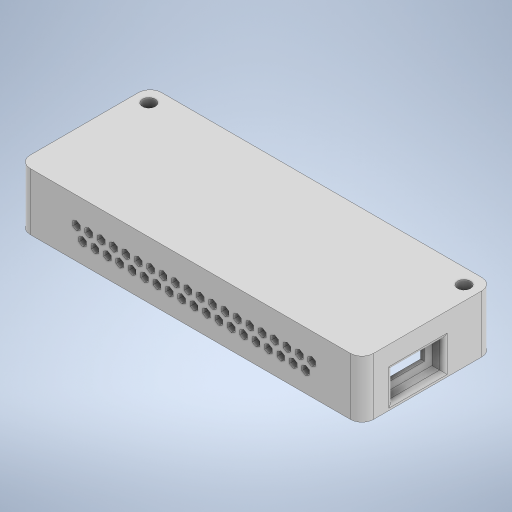
# Autodesk Inventor part: esp32_mount
Saved by Autodesk Inventor 2024 (Build 280153000, 153)
## iProperties
Created: 2024-01-28
Part Number: esp32_mount
Material: Generic
Document SubType Name: Modeling
Designer: crow
Density: 1 g/cm^3
Appearance: Default
Author: crow
## iProperties of the stored document esp32_mount_3DPrint.ipt
Created: 2024-01-28
Part Number: esp32_mount_3DPrint
Material: Generic
Document SubType Name: Modeling
Designer: crow
Density: 1 g/cm^3
Appearance: Default
Author: crow
Autodesk Inventor part; units mm, degrees
ref_plane "YZ Plane" through (0, 0, 0) normal (1, 0, 0) x (0, 1, 0)
ref_plane "XZ Plane" through (0, 0, 0) normal (0, 1, 0) x (-1, 0, 0)
ref_plane "XY Plane" through (0, 0, 0) normal (0, 0, 1) x (1, 0, 0)
sketch "Sketch1" plane through (0, 0, 0) normal (0, 1, 0) x (-1, 0, 0)
  line L0 (-0.1447, 76.4776) -> (-0.1447, -67.7737) construction
  line L1 (44.8553, -21.2084) -> (-45.1447, -21.2084)
  line L2 (-45.1447, -21.2084) -> (-45.1447, -13.2084)
  line L3 (-45.1447, -13.2084) -> (44.8553, -13.2084)
  line L4 (44.8553, -13.2084) -> (44.8553, -21.2084)
  line L5 (40.8553, 10.2416) -> (-41.1447, 10.2416)
  line L6 (-41.1447, 10.2416) -> (-41.1447, -13.2084)
  line L7 (-41.1447, -13.2084) -> (40.8553, -13.2084)
  line L8 (40.8553, -13.2084) -> (40.8553, 10.2416)
  circle A0 centre (8.6753, 7.4066) radius 1.25
  circle A1 centre (8.6753, -10.3734) radius 1.25
  circle A2 centre (-37.0447, -10.3734) radius 1.25
  line L9 (8.6753, 7.4066) -> (8.6753, -10.3734) construction
  line L10 (40.8553, -13.2084) -> (44.8553, -13.2084)
  line L11 (44.8553, -13.2084) -> (44.8553, 13.2416)
  line L12 (44.8553, 13.2416) -> (40.8553, 13.2416)
  line L13 (40.8553, 13.2416) -> (40.8553, -13.2084)
  line L14 (40.8553, 13.2416) -> (-45.1447, 13.2416)
  line L15 (-45.1447, 13.2416) -> (-45.1447, -13.2084)
  circle A3 centre (-37.0447, 7.4066) radius 1.25
  line L16 (-47.1247, -1.4834) -> (-6.1707, -1.4834) construction
  point P0 (0, 0)
  point P1 (41.1603, -17.2084)
  point P2 (-41.4497, -17.2084)
  point P3 (-0.1447, -13.2084)
  point P4 (8.6753, -1.4834)
  point P5 (40.8553, -13.2084)
  dimension "d0" = 82.61
  dimension "d1" = 41.305
  dimension "d2" = 90
  dimension "d3" = 8
  dimension "d4" = 4
  dimension "d5" = 3.695
  dimension "d6" = 82
  dimension "d7" = 23.45
  dimension "d10" = 2.5
  dimension "d11" = 17.78
  dimension "d16" = 43.22
  dimension "d17" = 4
  dimension "d18" = 3
  dimension "d19" = 4
  dimension "d82" = 2.5
  dimension "d85" = 4.1
  dimension "d86" = 45.72
  dimension "d87" = 17.78
  dimension "d91" = 11.725
  dimension "d92" = 8.89
  constraints: 34 end point, 6 parallel, 5 horizontal, 4 centre point, 4 perpendicular, 3 midpoint, 2 equal radius, 2 point on line, 2 vertical
  measures "d0" distance of point (41.16, -17.208) point (-41.45, -17.208)
  measures "d1" distance from line of L0 point (-41.45, -17.208)
  measures "d2" distance of L2.end L3.end
  measures "d3" distance of L1.end L2.end
  measures "d4" distance from line of L1 point (-41.45, -17.208)
  measures "d5" distance from line of L2 point (-41.45, -17.208)
  measures "d6" distance of L7.end L6.end
  measures "d7" distance of L6.end L5.end
  measures "d10" diameter of A0
  measures "d11" distance of L9.end L9.start
  measures "d17" distance of L12.end L11.end
  measures "d18" distance between parallel lines of L5 L12
  measures "d19" distance between parallel lines of L6 L15
  measures "d82" diameter of A3
  measures "d85" distance from line of L6 A3.centre
  measures "d86" distance of L9.start A3.centre
  measures "d87" distance of A2.centre A3.centre
  measures "d91" distance between parallel lines of L7 L16
  measures "d92" distance from line of L16 A2.centre
extrude "Extrusion1" add sketch "Sketch1" along normal blind 15 contours L1 L2 L3 L4 | L3 L8 L13 L12 L11 | L15 L14 L13 L5 L6 L3
sketch "Sketch2" plane through (0, 15, 0) normal (0, 1, 0) x (1, 0, 0)
  line L0 (-44.8553, 21.2084) -> (-44.8553, -13.2416) construction
  line L1 (45.1447, -13.2416) -> (45.1447, 21.2084) construction
  line L2 (50.5404, 17.2084) -> (-51.1103, 17.2084) construction
  point P0 (0, 0)
  point P1 (-41.1603, 17.2084)
  point P2 (41.4497, 17.2084)
  point P3 (-44.8553, 13.2084)
  point P4 (45.1447, 13.2084)
  dimension "d22" = 82.61
  dimension "d23" = 3.695
  constraints: 2 end point, 2 horizontal, 1 point on line
  measures "d22" distance of point (-41.16, 17.208) point (41.45, 17.208)
  measures "d23" distance from line of L1 point (41.45, 17.208)
hole "Hole1" at (-41.1603, 15, -17.2084) at (41.4497, 15, -17.2084) direction (0, -1, 0) diameter 3.4 depth 15 clearance for "Countersunk Flat Head Screw ISO 2009/7046" size "M3" standard "ISO"
sketch "Sketch3" plane through (0, 15, 0) normal (0, 1, 0) x (1, 0, 0)
  line L0 (45.1447, 21.2084) -> (-44.8553, 21.2084) projected
  line L1 (-40.8553, 13.2084) -> (41.1447, 13.2084) projected
  line L2 (-44.8553, 21.2084) -> (-29.4803, 21.2084)
  line L3 (-29.4803, 21.2084) -> (-29.4803, 13.2084)
  line L4 (-29.4803, 13.2084) -> (-44.8553, 13.2084)
  line L5 (-44.8553, 13.2084) -> (-44.8553, 21.2084)
  line L6 (-40.8553, 13.2084) -> (41.1447, 13.2084) projected
  line L7 (45.1447, -13.2416) -> (45.1447, 21.2084) projected
  line L8 (29.7697, 13.2084) -> (45.1447, 13.2084)
  line L9 (45.1447, 13.2084) -> (45.1447, 21.2084)
  line L10 (45.1447, 21.2084) -> (29.7697, 21.2084)
  line L11 (29.7697, 21.2084) -> (29.7697, 13.2084)
  circle A0 centre (-41.1603, 17.2084) radius 1.7 projected
  circle A1 centre (-41.1603, 17.2084) radius 3.1
  circle A2 centre (41.4497, 17.2084) radius 1.7 projected
  circle A3 centre (41.4497, 17.2084) radius 3.1
  point P0 (0, 0)
  point P1 (-44.8553, 13.2084)
  point P2 (45.1447, 13.2084)
  point P3 (-44.8553, 13.2084)
  point P4 (-40.8553, 5.069)
  point P5 (-40.8553, 2.0977)
  dimension "d72" = 1.4
  dimension "d73" = 1.4
  constraints: 16 end point, 4 parallel, 2 centre point, 2 coincident, 2 horizontal, 2 perpendicular, 1 other
  measures "d73" radial gap between concentric circles of A3 A2
extrude "Extrusion2" [suppressed]
sketch "Sketch4" plane through (0, 15, 0) normal (0, 1, 0) x (1, 0, 0)
  line L0 (41.1447, -10.2416) -> (-40.8553, -10.2416) projected
  line L1 (41.1447, 13.2084) -> (41.1447, -10.2416) projected
  line L2 (-40.8553, -10.2416) -> (41.1447, -10.2416)
  line L3 (41.1447, -10.2416) -> (41.1447, 13.2084)
  line L4 (41.1447, 13.2084) -> (-40.8553, 13.2084)
  line L5 (-40.8553, 13.2084) -> (-40.8553, -10.2416)
  point P0 (0, 0)
  constraints: 8 end point, 2 parallel, 1 horizontal, 1 perpendicular
extrude "Extrusion3" add sketch "Sketch4" against normal blind 2
sketch "Sketch5" plane through (0, 13, 0) normal (0, -1, 0) x (1, 0, 0)
  circle A0 centre (37.0447, -10.3734) radius 1.25 projected
  circle A1 centre (-8.6753, -10.3734) radius 1.25 projected
  circle A2 centre (-8.6753, 7.4066) radius 1.25 projected
  circle A3 centre (-8.6753, 7.4066) radius 2.5
  circle A4 centre (-8.6753, -10.3734) radius 2.5
  circle A5 centre (37.0447, -10.3734) radius 2.5
  circle A6 centre (37.0447, 7.4066) radius 1.25 projected
  circle A7 centre (37.0447, 7.4066) radius 2.5
  point P0 (0, 0)
  dimension "d35" = 5
  dimension "d36" = 5
  dimension "d37" = 5
  dimension "d83" = 5
  constraints: 4 centre point, 4 coincident
  measures "d35" diameter of A3
  measures "d36" diameter of A4
  measures "d37" diameter of A5
  measures "d83" diameter of A7
extrude "Extrusion4" add sketch "Sketch5" along normal blind 5 contours A0 | A1 | A2 | A3 | A4 | A5 | A6 | A7
sketch "Sketch6" plane through (37.0447, 8, -10.3734) normal (0, -1, 0) x (1, 0, 0)
  circle A0 centre (0, 0) radius 2.5 projected
  circle A1 centre (-45.72, 17.78) radius 2.5 projected
  circle A2 centre (-45.72, 0) radius 2.5 projected
  circle A3 centre (0, 17.78) radius 2.5 projected
  point P0 (-37.0447, 10.3734)
  point P1 (-45.72, 17.78)
  point P2 (-45.72, 0)
  point P3 (0, 17.78)
  constraints: 4 coincident
hole "Hole2" at (37.0447, 8, -10.3734) at (-8.6753, 8, 7.4066) at (-8.6753, 8, -10.3734) at (37.0447, 8, 7.4066) direction (0, 1, 0) diameter 2.4 depth 5
sketch "Sketch7" plane through (45.1447, 0, -14.0084) normal (-1, 0, 0) x (0, 0, 1)
  line L0 (7.885, 3.54) -> (17.225, 3.54)
  line L1 (17.225, 3.54) -> (17.225, 6.95)
  line L2 (17.225, 6.95) -> (7.885, 6.95)
  line L3 (7.885, 6.95) -> (7.885, 3.54)
  line L4 (0, 0) -> (27.25, 0) projected
  line L5 (0, 0) -> (0, 5) projected
  line L6 (27.25, 0) -> (27.25, 15) projected
  line L7 (0.8, 0) -> (0.8, 13) projected
  line L8 (27.25, 0) -> (-7.2, 0) projected
  point P0 (14.0084, 0)
  point P1 (24.25, 0)
  dimension "d53" = 6.95
  dimension "d56" = 7.025
  dimension "d88" = 7.085
  dimension "d89" = 3.54
  constraints: 8 end point, 2 parallel, 1 horizontal, 1 perpendicular, 1 other
  measures "d53" distance between parallel lines of L4 L2
  measures "d56" distance from line of point (24.25, 0) L1
  measures "d89" distance between parallel lines of L4 L0
extrude "Extrusion5" cut sketch "Sketch7" along normal blind 5
sketch "Sketch8" plane through (45.1447, 0, -14.0084) normal (-1, 0, 0) x (0, 0, 1)
  line L0 (5.885, 1.54) -> (19.225, 1.54)
  line L1 (19.225, 1.54) -> (19.225, 8.95)
  line L2 (19.225, 8.95) -> (5.885, 8.95)
  line L3 (5.885, 8.95) -> (5.885, 1.54)
  line L4 (7.885, 3.54) -> (17.225, 3.54) projected
  line L5 (7.885, 6.95) -> (7.885, 3.54) projected
  line L6 (17.225, 6.95) -> (7.885, 6.95) projected
  line L7 (17.225, 3.54) -> (17.225, 6.95) projected
  point P0 (14.0084, 0)
  dimension "d93" = 2
  dimension "d94" = 2
  dimension "d95" = 2
  dimension "d96" = 2
  constraints: 8 end point, 2 parallel, 1 horizontal, 1 perpendicular
  measures "d93" distance between parallel lines of L5 L3
  measures "d94" distance between parallel lines of L0 L4
  measures "d95" distance between parallel lines of L1 L7
  measures "d96" distance between parallel lines of L6 L2
extrude "Extrusion6" cut sketch "Sketch8" along normal blind 3 contours L3 L2 L1 L0 | L5 L6 L7 L4
fillet "Fillet2" radius 1 4 edges at (45.1447, 5.245, -8.1234) (45.1447, 1.54, -1.4534) (45.1447, 8.95, -1.4534) (45.1447, 5.245, 5.2166)
sketch "Sketch9" plane through (-44.8553, 0, 13.2416) normal (0, 0, 1) x (1, 0, 0)
  line L0 (39.5056, 7.1579) -> (41.1292, 6.2205)
  line L1 (41.1292, 6.2205) -> (41.1292, 4.3457)
  line L2 (41.1292, 4.3457) -> (39.5056, 3.4083)
  line L3 (39.5056, 3.4083) -> (37.882, 4.3457)
  line L4 (37.882, 4.3457) -> (37.882, 6.2205)
  line L5 (37.882, 6.2205) -> (39.5056, 7.1579)
  line L6 (39.5056, 7.1579) -> (39.5056, 9.0326)
  line L7 (39.5056, 9.0326) -> (37.882, 9.97)
  line L8 (37.882, 9.97) -> (36.2584, 9.0326)
  line L9 (36.2584, 9.0326) -> (36.2584, 7.1579)
  line L10 (36.2584, 7.1579) -> (37.882, 6.2205)
  line L11 (37.882, 6.2205) -> (37.882, 4.3457)
  line L12 (34.6348, 4.3457) -> (34.6348, 6.2205)
  line L13 (36.2584, 3.4083) -> (34.6348, 4.3457)
  line L14 (37.882, 4.3457) -> (36.2584, 3.4083)
  line L15 (34.6348, 6.2205) -> (36.2584, 7.1579)
  line L16 (34.6348, 9.97) -> (36.2584, 9.0326)
  line L17 (36.2584, 7.1579) -> (36.2584, 9.0326)
  line L18 (34.6348, 9.97) -> (33.0112, 9.0326)
  line L19 (33.0112, 9.0326) -> (33.0112, 7.1579)
  line L20 (33.0112, 7.1579) -> (34.6348, 6.2205)
  line L21 (33.0112, 3.4083) -> (34.6348, 4.3457)
  line L22 (34.6348, 6.2205) -> (34.6348, 4.3457)
  line L23 (31.3876, 4.3457) -> (31.3876, 6.2205)
  line L24 (31.3876, 4.3457) -> (33.0112, 3.4083)
  line L25 (31.3876, 6.2205) -> (33.0112, 7.1579)
  line L26 (31.3876, 9.97) -> (33.0112, 9.0326)
  line L27 (33.0112, 7.1579) -> (33.0112, 9.0326)
  line L28 (29.764, 7.1579) -> (29.764, 9.0326)
  line L29 (29.764, 7.1579) -> (31.3876, 6.2205)
  line L30 (29.764, 9.0326) -> (31.3876, 9.97)
  line L31 (39.5056, 6.4378) -> (40.5056, 5.8604)
  line L32 (40.5056, 5.8604) -> (40.5056, 4.7057)
  line L33 (40.5056, 4.7057) -> (39.5056, 4.1284)
  line L34 (39.5056, 4.1284) -> (38.5056, 4.7057)
  line L35 (38.5056, 4.7057) -> (38.5056, 5.8604)
  line L36 (38.5056, 5.8604) -> (39.5056, 6.4378)
  line L37 (36.2584, 6.4378) -> (35.2584, 5.8604)
  line L38 (35.2584, 5.8604) -> (35.2584, 4.7057)
  line L39 (35.2584, 4.7057) -> (36.2584, 4.1284)
  line L40 (36.2584, 4.1284) -> (37.2584, 4.7057)
  line L41 (37.2584, 4.7057) -> (37.2584, 5.8604)
  line L42 (37.2584, 5.8604) -> (36.2584, 6.4378)
  line L43 (33.0112, 6.4378) -> (34.0112, 5.8604)
  line L44 (32.0112, 5.8604) -> (33.0112, 6.4378)
  line L45 (32.0112, 4.7057) -> (32.0112, 5.8604)
  line L46 (34.0112, 5.8604) -> (34.0112, 4.7057)
  line L47 (34.0112, 4.7057) -> (33.0112, 4.1284)
  line L48 (33.0112, 4.1284) -> (32.0112, 4.7057)
  line L49 (33.6348, 8.6726) -> (33.6348, 7.5179)
  line L50 (33.6348, 7.5179) -> (34.6348, 6.9406)
  line L51 (34.6348, 9.25) -> (33.6348, 8.6726)
  line L52 (34.6348, 6.9406) -> (35.6348, 7.5179)
  line L53 (35.6348, 8.6726) -> (34.6348, 9.25)
  line L54 (35.6348, 7.5179) -> (35.6348, 8.6726)
  line L55 (32.3876, 8.6726) -> (32.3876, 7.5179)
  line L56 (32.3876, 7.5179) -> (31.3876, 6.9406)
  line L57 (31.3876, 9.25) -> (32.3876, 8.6726)
  line L58 (30.3876, 8.6726) -> (31.3876, 9.25)
  line L59 (31.3876, 6.9406) -> (30.3876, 7.5179)
  line L60 (30.3876, 7.5179) -> (30.3876, 8.6726)
  line L61 (38.882, 8.6726) -> (38.882, 7.5179)
  line L62 (38.882, 7.5179) -> (37.882, 6.9406)
  line L63 (37.882, 9.25) -> (38.882, 8.6726)
  line L64 (36.882, 8.6726) -> (37.882, 9.25)
  line L65 (37.882, 6.9406) -> (36.882, 7.5179)
  line L66 (36.882, 7.5179) -> (36.882, 8.6726)
  line L67 (41.1292, 6.2205) -> (42.7528, 7.1579)
  line L68 (42.7528, 7.1579) -> (42.7528, 9.0326)
  line L69 (42.7528, 9.0326) -> (41.1292, 9.97)
  line L70 (41.1292, 9.97) -> (39.5056, 9.0326)
  line L71 (39.5056, 9.0326) -> (39.5056, 7.1579)
  line L72 (40.1292, 7.5179) -> (41.1292, 6.9406)
  line L73 (41.1292, 6.9406) -> (42.1292, 7.5179)
  line L74 (42.1292, 7.5179) -> (42.1292, 8.6726)
  line L75 (42.1292, 8.6726) -> (41.1292, 9.25)
  line L76 (41.1292, 9.25) -> (40.1292, 8.6726)
  line L77 (40.1292, 8.6726) -> (40.1292, 7.5179)
  line L78 (41.1292, 4.3457) -> (41.1292, 6.2205)
  line L79 (41.1292, 4.3457) -> (42.7528, 3.4083)
  line L80 (42.7528, 4.1284) -> (41.7528, 4.7057)
  line L81 (43.7528, 4.7057) -> (42.7528, 4.1284)
  line L82 (43.7528, 5.8604) -> (43.7528, 4.7057)
  line L83 (44.3764, 6.2205) -> (44.3764, 4.3457)
  line L84 (42.7528, 6.4378) -> (43.7528, 5.8604)
  line L85 (41.7528, 5.8604) -> (42.7528, 6.4378)
  line L86 (41.7528, 4.7057) -> (41.7528, 5.8604)
  line L87 (42.7528, 7.1579) -> (44.3764, 6.2205)
  line L88 (44.3764, 4.3457) -> (42.7528, 3.4083)
  line L89 (42.7528, 9.0326) -> (44.3764, 9.97)
  line L90 (42.7528, 9.0326) -> (42.7528, 7.1579)
  line L91 (45.3764, 7.5179) -> (45.3764, 8.6726)
  line L92 (44.3764, 9.25) -> (43.3764, 8.6726)
  line L93 (44.3764, 6.9406) -> (45.3764, 7.5179)
  line L94 (43.3764, 8.6726) -> (43.3764, 7.5179)
  line L95 (43.3764, 7.5179) -> (44.3764, 6.9406)
  line L96 (44.3764, 6.2205) -> (46, 7.1579)
  line L97 (45.3764, 8.6726) -> (44.3764, 9.25)
  line L98 (44.3764, 9.97) -> (46, 9.0326)
  line L99 (46, 7.1579) -> (46, 9.0326)
  line L100 (90, 0) -> (90, 15) projected
  line L101 (23.2695, 7.1579) -> (24.8931, 6.2205)
  line L102 (24.8931, 6.2205) -> (24.8931, 4.3457)
  line L103 (24.8931, 4.3457) -> (23.2695, 3.4083)
  line L104 (23.2695, 3.4083) -> (21.6459, 4.3457)
  line L105 (21.6459, 4.3457) -> (21.6459, 6.2205)
  line L106 (21.6459, 6.2205) -> (23.2695, 7.1579)
  line L107 (21.6459, 9.97) -> (20.0223, 9.0326)
  line L108 (23.2695, 9.0326) -> (21.6459, 9.97)
  line L109 (23.2695, 7.1579) -> (23.2695, 9.0326)
  line L110 (20.0223, 7.1579) -> (21.6459, 6.2205)
  line L111 (20.0223, 9.0326) -> (20.0223, 7.1579)
  line L112 (21.6459, 4.3457) -> (20.0223, 3.4083)
  line L113 (20.0223, 3.4083) -> (18.3987, 4.3457)
  line L114 (18.3987, 4.3457) -> (18.3987, 6.2205)
  line L115 (18.3987, 6.2205) -> (20.0223, 7.1579)
  line L116 (21.6459, 6.2205) -> (21.6459, 4.3457)
  line L117 (18.3987, 9.97) -> (16.7751, 9.0326)
  line L118 (18.3987, 9.97) -> (20.0223, 9.0326)
  line L119 (20.0223, 7.1579) -> (20.0223, 9.0326)
  line L120 (16.7751, 7.1579) -> (18.3987, 6.2205)
  line L121 (16.7751, 9.0326) -> (16.7751, 7.1579)
  line L122 (15.1515, 4.3457) -> (16.7751, 3.4083)
  line L123 (15.1515, 4.3457) -> (15.1515, 6.2205)
  line L124 (15.1515, 6.2205) -> (16.7751, 7.1579)
  line L125 (18.3987, 6.2205) -> (18.3987, 4.3457)
  line L126 (16.7751, 3.4083) -> (18.3987, 4.3457)
  line L127 (16.7751, 7.1579) -> (16.7751, 9.0326)
  line L128 (13.5279, 9.0326) -> (15.1515, 9.97)
  line L129 (13.5279, 7.1579) -> (13.5279, 9.0326)
  line L130 (13.5279, 7.1579) -> (15.1515, 6.2205)
  line L131 (15.1515, 9.97) -> (16.7751, 9.0326)
  line L132 (23.2695, 6.4378) -> (24.2695, 5.8604)
  line L133 (24.2695, 5.8604) -> (24.2695, 4.7057)
  line L134 (24.2695, 4.7057) -> (23.2695, 4.1284)
  line L135 (23.2695, 4.1284) -> (22.2695, 4.7057)
  line L136 (22.2695, 4.7057) -> (22.2695, 5.8604)
  line L137 (22.2695, 5.8604) -> (23.2695, 6.4378)
  line L138 (20.0223, 6.4378) -> (19.0223, 5.8604)
  line L139 (21.0223, 5.8604) -> (20.0223, 6.4378)
  line L140 (21.0223, 4.7057) -> (21.0223, 5.8604)
  line L141 (19.0223, 5.8604) -> (19.0223, 4.7057)
  line L142 (19.0223, 4.7057) -> (20.0223, 4.1284)
  line L143 (20.0223, 4.1284) -> (21.0223, 4.7057)
  line L144 (15.7751, 5.8604) -> (16.7751, 6.4378)
  line L145 (16.7751, 6.4378) -> (17.7751, 5.8604)
  line L146 (15.7751, 4.7057) -> (15.7751, 5.8604)
  line L147 (17.7751, 5.8604) -> (17.7751, 4.7057)
  line L148 (16.7751, 4.1284) -> (15.7751, 4.7057)
  line L149 (17.7751, 4.7057) -> (16.7751, 4.1284)
  line L150 (17.3987, 8.6726) -> (17.3987, 7.5179)
  line L151 (17.3987, 7.5179) -> (18.3987, 6.9406)
  line L152 (18.3987, 9.25) -> (17.3987, 8.6726)
  line L153 (19.3987, 8.6726) -> (18.3987, 9.25)
  line L154 (18.3987, 6.9406) -> (19.3987, 7.5179)
  line L155 (19.3987, 7.5179) -> (19.3987, 8.6726)
  line L156 (16.1515, 7.5179) -> (15.1515, 6.9406)
  line L157 (15.1515, 6.9406) -> (14.1515, 7.5179)
  line L158 (16.1515, 8.6726) -> (16.1515, 7.5179)
  line L159 (15.1515, 9.25) -> (16.1515, 8.6726)
  line L160 (14.1515, 7.5179) -> (14.1515, 8.6726)
  line L161 (14.1515, 8.6726) -> (15.1515, 9.25)
  line L162 (22.6459, 7.5179) -> (21.6459, 6.9406)
  line L163 (21.6459, 6.9406) -> (20.6459, 7.5179)
  line L164 (22.6459, 8.6726) -> (22.6459, 7.5179)
  line L165 (21.6459, 9.25) -> (22.6459, 8.6726)
  line L166 (20.6459, 7.5179) -> (20.6459, 8.6726)
  line L167 (20.6459, 8.6726) -> (21.6459, 9.25)
  line L168 (23.8931, 8.6726) -> (23.8931, 7.5179)
  line L169 (23.2695, 9.0326) -> (23.2695, 7.1579)
  line L170 (24.8931, 9.25) -> (23.8931, 8.6726)
  line L171 (25.8931, 8.6726) -> (24.8931, 9.25)
  line L172 (26.5167, 9.0326) -> (24.8931, 9.97)
  line L173 (25.8931, 7.5179) -> (25.8931, 8.6726)
  line L174 (24.8931, 6.9406) -> (25.8931, 7.5179)
  line L175 (23.8931, 7.5179) -> (24.8931, 6.9406)
  line L176 (26.5167, 7.1579) -> (26.5167, 9.0326)
  line L177 (24.8931, 6.2205) -> (26.5167, 7.1579)
  line L178 (24.8931, 9.97) -> (23.2695, 9.0326)
  line L179 (27.5167, 4.7057) -> (26.5167, 4.1284)
  line L180 (25.5167, 4.7057) -> (25.5167, 5.8604)
  line L181 (27.5167, 5.8604) -> (27.5167, 4.7057)
  line L182 (25.5167, 5.8604) -> (26.5167, 6.4378)
  line L183 (26.5167, 6.4378) -> (27.5167, 5.8604)
  line L184 (28.1404, 6.2205) -> (28.1404, 4.3457)
  line L185 (26.5167, 7.1579) -> (28.1404, 6.2205)
  line L186 (26.5167, 4.1284) -> (25.5167, 4.7057)
  line L187 (24.8931, 4.3457) -> (26.5167, 3.4083)
  line L188 (28.1404, 4.3457) -> (26.5167, 3.4083)
  line L189 (24.8931, 4.3457) -> (24.8931, 6.2205)
  line L190 (26.5167, 9.0326) -> (26.5167, 7.1579)
  line L191 (27.1404, 8.6726) -> (27.1404, 7.5179)
  line L192 (27.1404, 7.5179) -> (28.1404, 6.9406)
  line L193 (29.1404, 8.6726) -> (28.1404, 9.25)
  line L194 (28.1404, 6.9406) -> (29.1404, 7.5179)
  line L195 (28.1404, 9.97) -> (29.764, 9.0326)
  line L196 (29.1404, 7.5179) -> (29.1404, 8.6726)
  line L197 (28.1404, 6.2205) -> (29.764, 7.1579)
  line L198 (29.764, 7.1579) -> (29.764, 9.0326)
  line L199 (26.5167, 9.0326) -> (28.1404, 9.97)
  line L200 (28.1404, 9.25) -> (27.1404, 8.6726)
  line L201 (28.1404, 4.3457) -> (28.1404, 6.2205)
  line L202 (29.764, 7.1579) -> (28.1404, 6.2205)
  line L203 (31.3876, 4.3457) -> (29.764, 3.4083)
  line L204 (31.3876, 6.2205) -> (29.764, 7.1579)
  line L205 (29.764, 3.4083) -> (28.1404, 4.3457)
  line L206 (33.0112, 7.1579) -> (31.3876, 6.2205)
  line L207 (30.764, 5.8604) -> (29.764, 6.4378)
  line L208 (29.764, 6.4378) -> (28.764, 5.8604)
  line L209 (30.764, 4.7057) -> (30.764, 5.8604)
  line L210 (28.764, 5.8604) -> (28.764, 4.7057)
  line L211 (29.764, 4.1284) -> (30.764, 4.7057)
  line L212 (28.764, 4.7057) -> (29.764, 4.1284)
  line L213 (71.9777, 7.1579) -> (73.6013, 6.2205)
  line L214 (73.6013, 6.2205) -> (73.6013, 4.3457)
  line L215 (73.6013, 4.3457) -> (71.9777, 3.4083)
  line L216 (71.9777, 3.4083) -> (70.3541, 4.3457)
  line L217 (70.3541, 4.3457) -> (70.3541, 6.2205)
  line L218 (70.3541, 6.2205) -> (71.9777, 7.1579)
  line L219 (70.3541, 9.97) -> (68.7305, 9.0326)
  line L220 (71.9777, 9.0326) -> (70.3541, 9.97)
  line L221 (71.9777, 7.1579) -> (71.9777, 9.0326)
  line L222 (68.7305, 7.1579) -> (70.3541, 6.2205)
  line L223 (68.7305, 9.0326) -> (68.7305, 7.1579)
  line L224 (70.3541, 4.3457) -> (68.7305, 3.4083)
  line L225 (68.7305, 3.4083) -> (67.1069, 4.3457)
  line L226 (67.1069, 4.3457) -> (67.1069, 6.2205)
  line L227 (67.1069, 6.2205) -> (68.7305, 7.1579)
  line L228 (70.3541, 6.2205) -> (70.3541, 4.3457)
  line L229 (67.1069, 9.97) -> (65.4833, 9.0326)
  line L230 (67.1069, 9.97) -> (68.7305, 9.0326)
  line L231 (68.7305, 7.1579) -> (68.7305, 9.0326)
  line L232 (65.4833, 7.1579) -> (67.1069, 6.2205)
  line L233 (65.4833, 9.0326) -> (65.4833, 7.1579)
  line L234 (63.8596, 4.3457) -> (65.4833, 3.4083)
  line L235 (63.8596, 4.3457) -> (63.8596, 6.2205)
  line L236 (63.8596, 6.2205) -> (65.4833, 7.1579)
  line L237 (67.1069, 6.2205) -> (67.1069, 4.3457)
  line L238 (65.4833, 3.4083) -> (67.1069, 4.3457)
  line L239 (65.4833, 7.1579) -> (65.4833, 9.0326)
  line L240 (62.236, 9.0326) -> (63.8596, 9.97)
  line L241 (62.236, 7.1579) -> (62.236, 9.0326)
  line L242 (62.236, 7.1579) -> (63.8596, 6.2205)
  line L243 (63.8596, 9.97) -> (65.4833, 9.0326)
  line L244 (71.9777, 6.4378) -> (72.9777, 5.8604)
  line L245 (72.9777, 5.8604) -> (72.9777, 4.7057)
  line L246 (72.9777, 4.7057) -> (71.9777, 4.1284)
  line L247 (71.9777, 4.1284) -> (70.9777, 4.7057)
  line L248 (70.9777, 4.7057) -> (70.9777, 5.8604)
  line L249 (70.9777, 5.8604) -> (71.9777, 6.4378)
  line L250 (68.7305, 6.4378) -> (67.7305, 5.8604)
  line L251 (69.7305, 5.8604) -> (68.7305, 6.4378)
  line L252 (69.7305, 4.7057) -> (69.7305, 5.8604)
  line L253 (67.7305, 5.8604) -> (67.7305, 4.7057)
  line L254 (67.7305, 4.7057) -> (68.7305, 4.1284)
  line L255 (68.7305, 4.1284) -> (69.7305, 4.7057)
  line L256 (64.4833, 5.8604) -> (65.4833, 6.4378)
  line L257 (65.4833, 6.4378) -> (66.4833, 5.8604)
  line L258 (64.4833, 4.7057) -> (64.4833, 5.8604)
  line L259 (66.4833, 5.8604) -> (66.4833, 4.7057)
  line L260 (65.4833, 4.1284) -> (64.4833, 4.7057)
  line L261 (66.4833, 4.7057) -> (65.4833, 4.1284)
  line L262 (66.1069, 8.6726) -> (66.1069, 7.5179)
  line L263 (66.1069, 7.5179) -> (67.1069, 6.9406)
  line L264 (67.1069, 9.25) -> (66.1069, 8.6726)
  line L265 (68.1069, 8.6726) -> (67.1069, 9.25)
  line L266 (67.1069, 6.9406) -> (68.1069, 7.5179)
  line L267 (68.1069, 7.5179) -> (68.1069, 8.6726)
  line L268 (64.8596, 7.5179) -> (63.8596, 6.9406)
  line L269 (63.8596, 6.9406) -> (62.8596, 7.5179)
  line L270 (64.8596, 8.6726) -> (64.8596, 7.5179)
  line L271 (63.8596, 9.25) -> (64.8596, 8.6726)
  line L272 (62.8596, 7.5179) -> (62.8596, 8.6726)
  line L273 (62.8596, 8.6726) -> (63.8596, 9.25)
  line L274 (71.3541, 7.5179) -> (70.3541, 6.9406)
  line L275 (70.3541, 6.9406) -> (69.3541, 7.5179)
  line L276 (71.3541, 8.6726) -> (71.3541, 7.5179)
  line L277 (70.3541, 9.25) -> (71.3541, 8.6726)
  line L278 (69.3541, 7.5179) -> (69.3541, 8.6726)
  line L279 (69.3541, 8.6726) -> (70.3541, 9.25)
  line L280 (72.6013, 8.6726) -> (72.6013, 7.5179)
  line L281 (71.9777, 9.0326) -> (71.9777, 7.1579)
  line L282 (73.6013, 9.25) -> (72.6013, 8.6726)
  line L283 (74.6013, 8.6726) -> (73.6013, 9.25)
  line L284 (75.2249, 9.0326) -> (73.6013, 9.97)
  line L285 (74.6013, 7.5179) -> (74.6013, 8.6726)
  line L286 (73.6013, 6.9406) -> (74.6013, 7.5179)
  line L287 (72.6013, 7.5179) -> (73.6013, 6.9406)
  line L288 (75.2249, 7.1579) -> (75.2249, 9.0326)
  line L289 (73.6013, 6.2205) -> (75.2249, 7.1579)
  line L290 (73.6013, 9.97) -> (71.9777, 9.0326)
  line L291 (76.2249, 4.7057) -> (75.2249, 4.1284)
  line L292 (74.2249, 4.7057) -> (74.2249, 5.8604)
  line L293 (76.2249, 5.8604) -> (76.2249, 4.7057)
  line L294 (74.2249, 5.8604) -> (75.2249, 6.4378)
  line L295 (75.2249, 6.4378) -> (76.2249, 5.8604)
  line L296 (76.8485, 6.2205) -> (76.8485, 4.3457)
  line L297 (75.2249, 7.1579) -> (76.8485, 6.2205)
  line L298 (75.2249, 4.1284) -> (74.2249, 4.7057)
  line L299 (73.6013, 4.3457) -> (75.2249, 3.4083)
  line L300 (76.8485, 4.3457) -> (75.2249, 3.4083)
  line L301 (73.6013, 4.3457) -> (73.6013, 6.2205)
  line L302 (75.2249, 9.0326) -> (75.2249, 7.1579)
  line L303 (75.8485, 8.6726) -> (75.8485, 7.5179)
  line L304 (75.8485, 7.5179) -> (76.8485, 6.9406)
  line L305 (77.8485, 8.6726) -> (76.8485, 9.25)
  line L306 (76.8485, 6.9406) -> (77.8485, 7.5179)
  line L307 (76.8485, 9.97) -> (78.4721, 9.0326)
  line L308 (77.8485, 7.5179) -> (77.8485, 8.6726)
  line L309 (76.8485, 6.2205) -> (78.4721, 7.1579)
  line L310 (78.4721, 7.1579) -> (78.4721, 9.0326)
  line L311 (75.2249, 9.0326) -> (76.8485, 9.97)
  line L312 (76.8485, 9.25) -> (75.8485, 8.6726)
  line L313 (55.7416, 7.1579) -> (57.3652, 6.2205)
  line L314 (57.3652, 6.2205) -> (57.3652, 4.3457)
  line L315 (57.3652, 4.3457) -> (55.7416, 3.4083)
  line L316 (55.7416, 3.4083) -> (54.118, 4.3457)
  line L317 (54.118, 4.3457) -> (54.118, 6.2205)
  line L318 (54.118, 6.2205) -> (55.7416, 7.1579)
  line L319 (54.7416, 5.8604) -> (55.7416, 6.4378)
  line L320 (55.7416, 6.4378) -> (56.7416, 5.8604)
  line L321 (54.7416, 4.7057) -> (54.7416, 5.8604)
  line L322 (55.7416, 4.1284) -> (54.7416, 4.7057)
  line L323 (56.7416, 5.8604) -> (56.7416, 4.7057)
  line L324 (56.7416, 4.7057) -> (55.7416, 4.1284)
  line L325 (54.118, 6.2205) -> (54.118, 4.3457)
  line L326 (52.4944, 7.1579) -> (54.118, 6.2205)
  line L327 (54.118, 4.3457) -> (52.4944, 3.4083)
  line L328 (52.4944, 3.4083) -> (50.8708, 4.3457)
  line L329 (50.8708, 4.3457) -> (50.8708, 6.2205)
  line L330 (50.8708, 6.2205) -> (52.4944, 7.1579)
  line L331 (52.4944, 6.4378) -> (51.4944, 5.8604)
  line L332 (53.4944, 5.8604) -> (52.4944, 6.4378)
  line L333 (51.4944, 5.8604) -> (51.4944, 4.7057)
  line L334 (50.8708, 6.2205) -> (50.8708, 4.3457)
  line L335 (51.4944, 4.7057) -> (52.4944, 4.1284)
  line L336 (53.4944, 4.7057) -> (53.4944, 5.8604)
  line L337 (52.4944, 4.1284) -> (53.4944, 4.7057)
  line L338 (49.2472, 9.0326) -> (49.2472, 7.1579)
  line L339 (47.6236, 6.2205) -> (49.2472, 7.1579)
  line L340 (49.2472, 7.1579) -> (49.2472, 9.0326)
  line L341 (46, 9.0326) -> (47.6236, 9.97)
  line L342 (48.6236, 7.5179) -> (47.6236, 6.9406)
  line L343 (48.6236, 8.6726) -> (48.6236, 7.5179)
  line L344 (47.6236, 6.9406) -> (46.6236, 7.5179)
  line L345 (46, 7.1579) -> (47.6236, 6.2205)
  line L346 (47.6236, 9.97) -> (49.2472, 9.0326)
  line L347 (47.6236, 9.25) -> (48.6236, 8.6726)
  line L348 (46.6236, 7.5179) -> (46.6236, 8.6726)
  line L349 (46.6236, 8.6726) -> (47.6236, 9.25)
  line L350 (46, 7.1579) -> (46, 9.0326)
  line L351 (52.4944, 9.0326) -> (52.4944, 7.1579)
  line L352 (50.8708, 9.97) -> (49.2472, 9.0326)
  line L353 (50.8708, 6.9406) -> (51.8708, 7.5179)
  line L354 (49.8708, 7.5179) -> (50.8708, 6.9406)
  line L355 (51.8708, 7.5179) -> (51.8708, 8.6726)
  line L356 (52.4944, 7.1579) -> (52.4944, 9.0326)
  line L357 (49.8708, 8.6726) -> (49.8708, 7.5179)
  line L358 (51.8708, 8.6726) -> (50.8708, 9.25)
  line L359 (50.8708, 9.25) -> (49.8708, 8.6726)
  line L360 (50.8708, 9.97) -> (52.4944, 9.0326)
  line L361 (55.118, 7.5179) -> (54.118, 6.9406)
  line L362 (54.118, 6.9406) -> (53.118, 7.5179)
  line L363 (55.118, 8.6726) -> (55.118, 7.5179)
  line L364 (55.7416, 7.1579) -> (55.7416, 9.0326)
  line L365 (53.118, 7.5179) -> (53.118, 8.6726)
  line L366 (54.118, 9.25) -> (55.118, 8.6726)
  line L367 (53.118, 8.6726) -> (54.118, 9.25)
  line L368 (54.118, 9.97) -> (52.4944, 9.0326)
  line L369 (55.7416, 9.0326) -> (54.118, 9.97)
  line L370 (49.2472, 7.1579) -> (50.8708, 6.2205)
  line L371 (47.6236, 4.3457) -> (49.2472, 3.4083)
  line L372 (47.6236, 4.3457) -> (47.6236, 6.2205)
  line L373 (49.2472, 3.4083) -> (50.8708, 4.3457)
  line L374 (48.2472, 5.8604) -> (49.2472, 6.4378)
  line L375 (49.2472, 6.4378) -> (50.2472, 5.8604)
  line L376 (48.2472, 4.7057) -> (48.2472, 5.8604)
  line L377 (49.2472, 4.1284) -> (48.2472, 4.7057)
  line L378 (50.2472, 5.8604) -> (50.2472, 4.7057)
  line L379 (50.2472, 4.7057) -> (49.2472, 4.1284)
  line L380 (55.7416, 9.0326) -> (55.7416, 7.1579)
  line L381 (56.3652, 8.6726) -> (56.3652, 7.5179)
  line L382 (57.3652, 9.25) -> (56.3652, 8.6726)
  line L383 (56.3652, 7.5179) -> (57.3652, 6.9406)
  line L384 (58.3652, 7.5179) -> (58.3652, 8.6726)
  line L385 (58.3652, 8.6726) -> (57.3652, 9.25)
  line L386 (57.3652, 6.9406) -> (58.3652, 7.5179)
  line L387 (57.3652, 6.2205) -> (58.9888, 7.1579)
  line L388 (58.9888, 7.1579) -> (58.9888, 9.0326)
  line L389 (58.9888, 9.0326) -> (58.9888, 7.1579)
  line L390 (58.9888, 9.0326) -> (57.3652, 9.97)
  line L391 (57.3652, 9.97) -> (55.7416, 9.0326)
  line L392 (59.9888, 4.7057) -> (58.9888, 4.1284)
  line L393 (57.9888, 4.7057) -> (57.9888, 5.8604)
  line L394 (59.9888, 5.8604) -> (59.9888, 4.7057)
  line L395 (58.9888, 6.4378) -> (59.9888, 5.8604)
  line L396 (60.6124, 6.2205) -> (60.6124, 4.3457)
  line L397 (60.6124, 4.3457) -> (58.9888, 3.4083)
  line L398 (58.9888, 4.1284) -> (57.9888, 4.7057)
  line L399 (57.3652, 4.3457) -> (57.3652, 6.2205)
  line L400 (57.3652, 4.3457) -> (58.9888, 3.4083)
  line L401 (57.9888, 5.8604) -> (58.9888, 6.4378)
  line L402 (59.6124, 8.6726) -> (59.6124, 7.5179)
  line L403 (60.6124, 9.25) -> (59.6124, 8.6726)
  line L404 (58.9888, 9.0326) -> (60.6124, 9.97)
  line L405 (59.6124, 7.5179) -> (60.6124, 6.9406)
  line L406 (58.9888, 7.1579) -> (60.6124, 6.2205)
  line L407 (61.6124, 8.6726) -> (60.6124, 9.25)
  line L408 (60.6124, 9.97) -> (62.236, 9.0326)
  line L409 (61.6124, 7.5179) -> (61.6124, 8.6726)
  line L410 (62.236, 7.1579) -> (62.236, 9.0326)
  line L411 (60.6124, 6.2205) -> (62.236, 7.1579)
  line L412 (60.6124, 6.9406) -> (61.6124, 7.5179)
  line L413 (63.236, 4.7057) -> (63.236, 5.8604)
  line L414 (61.236, 5.8604) -> (61.236, 4.7057)
  line L415 (61.236, 4.7057) -> (62.236, 4.1284)
  line L416 (62.236, 3.4083) -> (60.6124, 4.3457)
  line L417 (63.8596, 4.3457) -> (62.236, 3.4083)
  line L418 (62.236, 4.1284) -> (63.236, 4.7057)
  line L419 (65.4833, 7.1579) -> (63.8596, 6.2205)
  line L420 (62.236, 7.1579) -> (60.6124, 6.2205)
  line L421 (63.236, 5.8604) -> (62.236, 6.4378)
  line L422 (62.236, 6.4378) -> (61.236, 5.8604)
  line L423 (63.8596, 6.2205) -> (62.236, 7.1579)
  line L424 (60.6124, 4.3457) -> (60.6124, 6.2205)
  line L425 (44.3764, 6.2205) -> (44.3764, 4.3457)
  line L426 (47, 4.7057) -> (47, 5.8604)
  line L427 (46, 4.1284) -> (47, 4.7057)
  line L428 (47, 5.8604) -> (46, 6.4378)
  line L429 (45, 4.7057) -> (46, 4.1284)
  line L430 (44.3764, 4.3457) -> (46, 3.4083)
  line L431 (46, 6.4378) -> (45, 5.8604)
  line L432 (46, 7.1579) -> (44.3764, 6.2205)
  line L433 (45, 5.8604) -> (45, 4.7057)
  line L434 (46, 3.4083) -> (47.6236, 4.3457)
  line L435 (47.6236, 6.2205) -> (47.6236, 4.3457)
  point P0 (44.8553, 0)
  point P1 (39.5056, 5.2831)
  point P2 (39.5056, 5.2831)
  point P3 (36.2584, 5.2831)
  point P4 (36.2584, 5.2831)
  point P5 (33.0112, 5.2831)
  point P6 (33.0112, 5.2831)
  point P7 (34.6348, 8.0953)
  point P8 (34.6348, 8.0953)
  point P9 (31.3876, 8.0953)
  point P10 (31.3876, 8.0953)
  point P11 (37.882, 8.0953)
  point P12 (37.882, 8.0953)
  point P13 (31.3876, 5.2831)
  point P14 (41.1292, 8.0953)
  point P15 (41.1292, 8.0953)
  point P16 (42.7528, 5.2831)
  point P17 (42.7528, 5.2831)
  point P18 (44.3764, 8.0953)
  point P19 (44.3764, 8.0953)
  point P20 (43.7528, 5.2831)
  point P21 (23.2695, 5.2831)
  point P22 (23.2695, 5.2831)
  point P23 (20.0223, 5.2831)
  point P24 (20.0223, 5.2831)
  point P25 (16.7751, 5.2831)
  point P26 (16.7751, 5.2831)
  point P27 (18.3987, 8.0953)
  point P28 (18.3987, 8.0953)
  point P29 (15.1515, 8.0953)
  point P30 (15.1515, 8.0953)
  point P31 (21.6459, 8.0953)
  point P32 (21.6459, 8.0953)
  point P33 (15.1515, 5.2831)
  point P34 (24.8931, 8.0953)
  point P35 (24.8931, 8.0953)
  point P36 (26.5167, 5.2831)
  point P37 (26.5167, 5.2831)
  point P38 (28.1404, 8.0953)
  point P39 (28.1404, 8.0953)
  point P40 (27.5167, 5.2831)
  point P41 (29.764, 5.2831)
  point P42 (29.764, 5.2831)
  point P43 (71.9777, 5.2831)
  point P44 (71.9777, 5.2831)
  point P45 (68.7305, 5.2831)
  point P46 (68.7305, 5.2831)
  point P47 (65.4833, 5.2831)
  point P48 (65.4833, 5.2831)
  point P49 (67.1069, 8.0953)
  point P50 (67.1069, 8.0953)
  point P51 (63.8596, 8.0953)
  point P52 (63.8596, 8.0953)
  point P53 (70.3541, 8.0953)
  point P54 (70.3541, 8.0953)
  point P55 (63.8596, 5.2831)
  point P56 (73.6013, 8.0953)
  point P57 (73.6013, 8.0953)
  point P58 (75.2249, 5.2831)
  point P59 (75.2249, 5.2831)
  point P60 (76.8485, 8.0953)
  point P61 (76.8485, 8.0953)
  point P62 (76.2249, 5.2831)
  point P63 (55.7416, 5.2831)
  point P64 (55.7416, 5.2831)
  point P65 (52.4944, 5.2831)
  point P66 (52.4944, 5.2831)
  point P67 (47.6236, 8.0953)
  point P68 (47.6236, 8.0953)
  point P69 (50.8708, 8.0953)
  point P70 (50.8708, 8.0953)
  point P71 (54.118, 8.0953)
  point P72 (54.118, 8.0953)
  point P73 (47.6236, 5.2831)
  point P74 (49.2472, 5.2831)
  point P75 (49.2472, 5.2831)
  point P76 (57.3652, 8.0953)
  point P77 (57.3652, 8.0953)
  point P78 (58.9888, 5.2831)
  point P79 (58.9888, 5.2831)
  point P80 (59.9888, 5.2831)
  point P81 (60.6124, 8.0953)
  point P82 (60.6124, 8.0953)
  point P83 (62.236, 5.2831)
  point P84 (62.236, 5.2831)
  point P85 (46, 5.2831)
  point P86 (44.3764, 5.2831)
  point P87 (44.3764, 5.2831)
  dimension "d68" = 2
  dimension "d69" = 3.2472
  dimension "d74" = 44
  dimension "d76" = 2
  dimension "d77" = 3.2472
  dimension "d79" = 0
  dimension "d80" = 0
  dimension "d97" = 2
  dimension "d98" = 3.2472
  dimension "d99" = 2
  dimension "d100" = 3.2472
  dimension "d101" = 0
  dimension "d102" = 0
  dimension "d105" = 0
  constraints: 870 end point, 388 symmetric about line, 38 coincident, 10 midpoint, 104 other
  measures "d68" distance from line of point (43.753, 5.283) L86
  measures "d69" distance between parallel lines of L1 L83
  measures "d74" distance between parallel lines of L100 L99
  measures "d76" distance from line of point (27.517, 5.283) L180
  measures "d77" distance between parallel lines of L102 L184
  measures "d79" distance between parallel lines of L28 L198
  measures "d80" distance of L30.start L195.end
  measures "d97" distance from line of point (76.225, 5.283) L292
  measures "d98" distance between parallel lines of L214 L296
  measures "d99" distance from line of point (59.989, 5.283) L393
  measures "d100" distance between parallel lines of L314 L396
  measures "d101" distance between parallel lines of L241 L410
  measures "d102" distance of L241.end L408.end
  measures "d105" distance of point (44.376, 5.283) point (44.376, 5.283)
extrude "Extrusion7" cut sketch "Sketch9" against normal up to surface (3 mm away) contours L31 L32 L33 L34 L35 L36 | L42 L41 L40 L39 L38 L37 | L43 L46 L47 L48 L45 L44 | L51 L53 L54 L52 L50 L49 | L55 L56 L59 L60 L58 L57 | L61 L62 L65 L66 L64 L63 | L77 L76 L75 L74 L73 L72 | L80 L86 L85 L84 L82 L81 | L93 L95 L94 L92 L97 L91 | L132 L133 L134 L135 L136 L137 | L139 L140 L143 L142 L141 L138 | L144 L145 L147 L149 L148 L146 | L152 L153 L155 L154 L151 L150 | L156 L157 L160 L161 L159 L158 | L162 L163 L166 L167 L165 L164 | L170 L171 L173 L174 L175 L168 | L179 L186 L180 L182 L183 L181 | L200 L193 L196 L194 L192 L191 | L209 L211 L212 L210 L208 L207 | L244 L245 L246 L247 L248 L249 | L251 L252 L255 L254 L253 L250 | L256 L257 L259 L261 L260 L258 | L264 L265 L267 L266 L263 L262 | L268 L269 L272 L273 L271 L270 | L274 L275 L278 L279 L277 L276 | L282 L283 L285 L286 L287 L280 | L291 L298 L292 L294 L295 L293 | L312 L305 L308 L306 L304 L303 | L319 L320 L323 L324 L322 L321 | L332 L336 L337 L335 L333 L331 | L342 L344 L348 L349 L347 L343 | L354 L357 L359 L358 L355 L353 | L361 L362 L365 L367 L366 L363 | L374 L375 L378 L379 L377 L376 | L382 L385 L384 L386 L383 L381 | L392 L398 L393 L401 L395 L394 | L403 L407 L409 L412 L405 L402 | L418 L415 L414 L422 L421 L413 | L427 L429 L433 L431 L428 L426
fillet "Fillet3" radius 3 4 edges at (45.1447, 7.5, -21.2084) (45.1447, 7.5, 13.2416) (-44.8553, 7.5, 13.2416) (-44.8553, 7.5, -21.2084)
equation "\"d91\" = 0.5 * d7"
equation "\"d92\" = 0.5 * d11"
equation "\"d73\" = d72"
equation "\"d36\" = d35"
equation "\"d37\" = d35"
equation "\"d83\" = d35"
equation "\"d94\" = d93"
equation "\"d95\" = d93"
equation "\"d96\" = d93"
body "Solid189"
